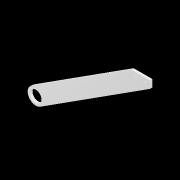
# Autodesk Inventor part: winch_support_starboard_forward
Saved by Autodesk Inventor 2020.2 (Build 242310000, 310)
## iProperties
Created: 2020-03-28
Part Number: winch_support_starboard_forward
Material: Aluminum 6061
Document SubType Name: Modeling
Designer: agmle
Density: 2.7 g/cm^3
Appearance: Aluminum - Flat
Mass: 241.575 g
Surface Area: 338.486 cm^2
Volume: 89.4721 cm^3
Author: agmle
Autodesk Inventor part; units mm, degrees
ref_plane "YZ Plane" through (0, 0, 0) normal (1, 0, 0) x (0, 1, 0)
ref_plane "XZ Plane" through (0, 0, 0) normal (0, 1, 0) x (-1, 0, 0)
ref_plane "XY Plane" through (0, 0, 0) normal (0, 0, 1) x (1, 0, 0)
sketch "Sketch1" plane through (0, 0, 0) normal (0, 0, 1) x (1, 0, 0)
  line L0 (-245.3259, 0) -> (63.2798, 244.4632) construction
  line L1 (63.2798, 244.4632) -> (245.3259, 0) construction
  line L2 (245.3259, 0) -> (-245.3259, 0) construction
  circle A0 centre (-245.3259, 0) radius 14.7955 construction
  circle A1 centre (245.3259, 0) radius 14.7955 construction
  arc A2 (-256.7323, 17.8052) -> (-233.9195, -17.8052) centre (-245.3259, 0) ccw
  arc A3 (228.3663, -12.6295) -> (262.2855, 12.6295) centre (245.3259, 0) ccw construction
  line L3 (-256.7323, 17.8052) -> (1.819, 183.4388)
  line L4 (1.819, 183.4388) -> (135.0877, 183.4388) construction
  line L5 (135.0877, 183.4388) -> (262.2855, 12.6295) construction
  line L6 (228.3663, -12.6295) -> (96.5448, 164.3888) construction
  line L7 (96.5448, 164.3888) -> (50.4824, 164.3888) construction
  line L8 (50.4824, 164.3888) -> (-233.9195, -17.8052)
  line L9 (50.4824, 183.4388) -> (1.819, 183.4388)
  line L10 (63.2798, 173.902) -> (13.7498, 173.902) construction
  line L11 (13.7498, 173.902) -> (5.9464, 186.0829) construction
  line L12 (38.5148, 173.902) -> (46.3181, 161.7211) construction
  line L13 (50.4824, 183.4388) -> (50.4824, 164.3888)
  line L14 (63.2798, 244.4632) -> (63.2798, 173.902) construction
  point P0 (0, 0)
  point P1 (0, 0)
  dimension "d0" = 304.8
  dimension "d1" = 393.7
  dimension "d2" = 490.6518
  dimension "d3" = 29.591
  dimension "d4" = 6.35
  dimension "d5" = 19.05
  dimension "d6" = 164.3888
  dimension "d36" = 49.53
  dimension "d37" = 70.5612
  constraints: 30 end point, 6 coincident, 5 parallel, 4 centre point, 4 point on circle, 4 tangent, 3 horizontal, 3 perpendicular, 3 point on line, 2 equal radius, 2 midpoint, 1 collinear, 1 vertical
  measures "d0" distance of L0.end L1.end
  measures "d1" distance of L0.start L0.end
  measures "d2" distance of L1.end L0.start
  measures "d3" diameter of A0
  measures "d4" radial gap between concentric circles of A0 A2
  measures "d5" distance between parallel lines of L7 L4
  measures "d6" distance between parallel lines of L2 L7
  measures "d36" distance of L10.start L10.end
  measures "d37" distance from line of L0.end L10
extrude "Frame" add sketch "Sketch1" along normal blind 6.35
sketch "Sketch2" plane through (0, 0, 6.35) normal (0, 0, 1) x (1, 0, 0)
  arc A0 (-256.7323, 17.8052) -> (-233.9195, -17.8052) centre (-245.3259, 0) ccw projected
  point P0 (0, 0)
  point P1 (-245.3259, 0)
  constraints: 1 coincident
hole "Struts" at (-245.3259, 0, 6.35) direction (0, 0, -1) diameter 29.591 end through all
fillet "Edge Break" radius 5 1 edges at (1.819, 183.4388, 3.175)
sketch "Sketch3" plane through (0, 0, 0) normal (0, 0, -1) x (-1, 0, 0)
  line L0 (-50.4824, 164.3888) -> (-50.4824, 183.4388) construction
  line L1 (233.9195, -17.8052) -> (-50.4824, 164.3888) construction
  line L2 (-0.5861, 182.649) -> (256.7323, 17.8052) construction
  line L3 (-38.5332, 173.9138) -> (-13.7682, 173.9138) construction
  line L4 (-13.7682, 173.9138) -> (-5.9649, 186.0947) construction
  line L5 (-0.5861, 182.649) -> (256.7323, 17.8052) construction
  line L6 (-38.5332, 173.9138) -> (-46.3366, 161.7329) construction
  point P0 (0, 0)
  point P1 (-50.4824, 173.9138)
  dimension "d33" = 24.765
  constraints: 6 end point, 3 point on line, 2 perpendicular, 1 coincident, 1 horizontal, 1 midpoint, 1 parallel
  measures "d33" distance of point (-38.533, 173.914) L3.end
hole "Mount Bolts" at (13.7682, 173.9138, 0) at (38.5332, 173.9138, 0) direction (0, 0, 1) diameter 3.4036 end through all countersink diameter 6.2992 countersink angle 90 clearance for "Flat Head Machine Screw" size "M3" standard "Ansi Metric M Profile"
body "Solid1"
